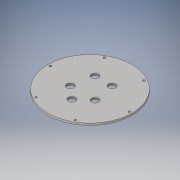
# Autodesk Inventor part: Back Lens
Saved by Autodesk Inventor 2016 (Build 200138000, 138)
## iProperties
Created: 2017-10-13
Part Number: Back Lens
Material: Generic
Document SubType Name: Modeling
Designer: Student
Density: 1 g/cm^3
Appearance: Default
Author: Student
Autodesk Inventor part; units mm, degrees
ref_plane "YZ Plane" through (0, 0, 0) normal (1, 0, 0) x (0, 1, 0)
ref_plane "XZ Plane" through (0, 0, 0) normal (0, 1, 0) x (-1, 0, 0)
ref_plane "XY Plane" through (0, 0, 0) normal (0, 0, 1) x (1, 0, 0)
sketch "Sketch1" plane through (0, 0, 0) normal (0, 1, 0) x (-1, 0, 0)
  circle A0 centre (0, 0) radius 58.801
  circle A1 centre (55.245, 0) radius 1.5
  circle A2 centre (27.6225, 47.8436) radius 1.5
  circle A3 centre (-27.6225, 47.8436) radius 1.5
  circle A4 centre (-55.245, 0) radius 1.5
  circle A5 centre (-27.6225, -47.8436) radius 1.5
  circle A6 centre (27.6225, -47.8436) radius 1.5
  dimension "d0" = 117.602
  dimension "d1" = 3
  dimension "d2" = 55.245
  dimension "d5" = 360
  constraints: 7 centre point, 1 coincident, 13 other
  measures "d0" diameter of A0
  measures "d1" diameter of A1
  measures "d2" distance of A1.centre point (0, 0)
extrude "Extrusion1" add sketch "Sketch1" along normal blind 2.7432
sketch "Sketch2" plane through (0, 2.7432, 0) normal (0, 1, 0) x (1, 0, 0)
  circle A0 centre (11.938, 18.9738) radius 4.9911
  circle A1 centre (-11.938, 18.9738) radius 4.9911
  circle A2 centre (17.272, -10.16) radius 4.9911
  circle A3 centre (-17.272, -10.16) radius 4.9911
  circle A4 centre (0, -25.4) radius 4.9911
  point P0 (0, 0)
  dimension "d9" = 9.9822
  dimension "d10" = 9.9822
  dimension "d11" = 11.938
  dimension "d12" = 11.938
  dimension "d13" = 18.9738
  dimension "d14" = 18.9738
  dimension "d15" = 25.4
  dimension "d16" = 10.16
  dimension "d17" = 10.16
  dimension "d18" = 9.9822
  dimension "d19" = 9.9822
  dimension "d20" = 9.9822
  dimension "d21" = 17.272
  dimension "d22" = 17.272
  constraints: 5 centre point
  measures "d9" diameter of A0
  measures "d10" diameter of A1
  measures "d11" horizontal distance of point (0, 0) A0.centre
  measures "d12" horizontal distance of A1.centre point (0, 0)
  measures "d13" vertical distance of A0.centre point (0, 0)
  measures "d14" vertical distance of A1.centre point (0, 0)
  measures "d15" distance of point (0, 0) A4.centre
  measures "d16" vertical distance of point (0, 0) A2.centre
  measures "d17" vertical distance of point (0, 0) A3.centre
  measures "d18" diameter of A3
  measures "d19" diameter of A2
  measures "d20" diameter of A4
  measures "d21" horizontal distance of point (0, 0) A2.centre
  measures "d22" horizontal distance of A3.centre point (0, 0)
extrude "Extrusion2" cut sketch "Sketch2" against normal blind 2.7432
equation "\"d14\" = d13"
body "Solid1"
